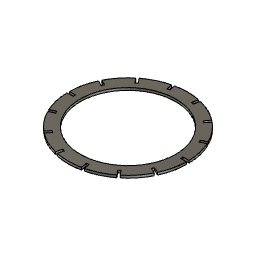
Hringur_Stor (Autodesk Fusion 360 design; units mm, degrees)
Autodesk Fusion 360 part; units mm, degrees
sketch "Sketch1" plane through (0, 0, 0) normal (0, 0, 1) x (1, 0, 0)
  circle A0 centre (0, 0) radius 80
  line L0 (99.98, 2) -> (89.98, 2)
  line L1 (89.98, 2) -> (89.98, -2)
  line L2 (89.98, -2) -> (99.98, -2)
  line L3 (89.2111, 45.1816) -> (80.2014, 40.8428)
  line L4 (81.9369, 37.2389) -> (90.9466, 41.5778)
  line L5 (80.2014, 40.8428) -> (81.9369, 37.2389)
  line L6 (60.7728, 79.4145) -> (54.5379, 71.5962)
  line L7 (57.6653, 69.1022) -> (63.9002, 76.9205)
  line L8 (54.5379, 71.5962) -> (57.6653, 69.1022)
  line L9 (20.2978, 97.9183) -> (18.0726, 88.1691)
  line L10 (21.9723, 87.279) -> (24.1975, 97.0282)
  line L11 (18.0726, 88.1691) -> (21.9723, 87.279)
  line L12 (-24.1975, 97.0282) -> (-21.9723, 87.279)
  line L13 (-18.0726, 88.1691) -> (-20.2978, 97.9183)
  line L14 (-21.9723, 87.279) -> (-18.0726, 88.1691)
  line L15 (-63.9002, 76.9205) -> (-57.6653, 69.1022)
  line L16 (-54.5379, 71.5962) -> (-60.7728, 79.4145)
  line L17 (-57.6653, 69.1022) -> (-54.5379, 71.5962)
  line L18 (-90.9466, 41.5778) -> (-81.9369, 37.2389)
  line L19 (-80.2014, 40.8428) -> (-89.2111, 45.1816)
  line L20 (-81.9369, 37.2389) -> (-80.2014, 40.8428)
  line L21 (-99.98, -2) -> (-89.98, -2)
  line L22 (-89.98, 2) -> (-99.98, 2)
  line L23 (-89.98, -2) -> (-89.98, 2)
  line L24 (-89.2111, -45.1816) -> (-80.2014, -40.8428)
  line L25 (-81.9369, -37.2389) -> (-90.9466, -41.5778)
  line L26 (-80.2014, -40.8428) -> (-81.9369, -37.2389)
  line L27 (-60.7728, -79.4145) -> (-54.5379, -71.5962)
  line L28 (-57.6653, -69.1022) -> (-63.9002, -76.9205)
  line L29 (-54.5379, -71.5962) -> (-57.6653, -69.1022)
  line L30 (-20.2978, -97.9183) -> (-18.0726, -88.1691)
  line L31 (-21.9723, -87.279) -> (-24.1975, -97.0282)
  line L32 (-18.0726, -88.1691) -> (-21.9723, -87.279)
  line L33 (24.1975, -97.0282) -> (21.9723, -87.279)
  line L34 (18.0726, -88.1691) -> (20.2978, -97.9183)
  line L35 (21.9723, -87.279) -> (18.0726, -88.1691)
  line L36 (63.9002, -76.9205) -> (57.6653, -69.1022)
  line L37 (54.5379, -71.5962) -> (60.7728, -79.4145)
  line L38 (57.6653, -69.1022) -> (54.5379, -71.5962)
  line L39 (90.9466, -41.5778) -> (81.9369, -37.2389)
  line L40 (80.2014, -40.8428) -> (89.2111, -45.1816)
  line L41 (81.9369, -37.2389) -> (80.2014, -40.8428)
  arc A1 (99.98, 2) -> (90.9466, 41.5778) centre (0, 0) ccw
  arc A2 (89.2111, 45.1816) -> (63.9002, 76.9205) centre (0, 0) ccw
  arc A3 (60.7728, 79.4145) -> (24.1975, 97.0282) centre (0, 0) ccw
  arc A4 (20.2978, 97.9183) -> (-20.2978, 97.9183) centre (0, 0) ccw
  arc A5 (-24.1975, 97.0282) -> (-60.7728, 79.4145) centre (0, 0) ccw
  arc A6 (-63.9002, 76.9205) -> (-89.2111, 45.1816) centre (0, 0) ccw
  arc A7 (-90.9466, 41.5778) -> (-99.98, 2) centre (0, 0) ccw
  arc A8 (-99.98, -2) -> (-90.9466, -41.5778) centre (0, 0) ccw
  arc A9 (-89.2111, -45.1816) -> (-63.9002, -76.9205) centre (0, 0) ccw
  arc A10 (90.9466, -41.5778) -> (99.98, -2) centre (0, 0) ccw
  arc A11 (63.9002, -76.9205) -> (89.2111, -45.1816) centre (0, 0) ccw
  arc A12 (24.1975, -97.0282) -> (60.7728, -79.4145) centre (0, 0) ccw
  arc A13 (-60.7728, -79.4145) -> (-24.1975, -97.0282) centre (0, 0) ccw
  arc A14 (-20.2978, -97.9183) -> (20.2978, -97.9183) centre (0, 0) ccw
  dimension "d1" = 200
  dimension "d2" = 160
  dimension "d5" = 4
  dimension "d6" = 10
  dimension "d7" = 10
  dimension "d13" = 360
  constraint coincident A0.centre A1.centre
  constraint horizontal L0
  constraint perpendicular L0 L1
  constraint perpendicular L1 L2
  constraint concentric A1 A2
  constraint concentric A2 A3
  constraint concentric A3 A4
  constraint concentric A4 A5
  constraint concentric A5 A6
  constraint concentric A6 A7
  constraint concentric A7 A8
  constraint concentric A8 A9
  constraint concentric A9 A13
  constraint concentric A10 A13
  constraint concentric A11 A13
  constraint concentric A12 A13
  constraint concentric A13 A14
  measures "d1" diameter of A1
  measures "d2" diameter of A0
  measures "d5" distance of L0.end L1.end
  measures "d6" distance of L0.start L0.end
  measures "d7" distance of L1.end L2.end
extrude "Extrude1" add sketch "Sketch1" along normal blind 4
component "Hringur_Stor" placed x (1, 0, 0) y (0, 1, 0) z (0, 0, 1) at (0, 0, 0)
equation "d1 = D_o"
equation "d2 = D_i"
equation "d5 = þykkt"
equation "d6 = dypt_pressfit"
equation "d7 = dypt_pressfit"
equation "D_o = 200 mm"
equation "D_i = 160 mm"
equation "dypt_pressfit = 10 mm"
equation "þykkt = 4 mm"
